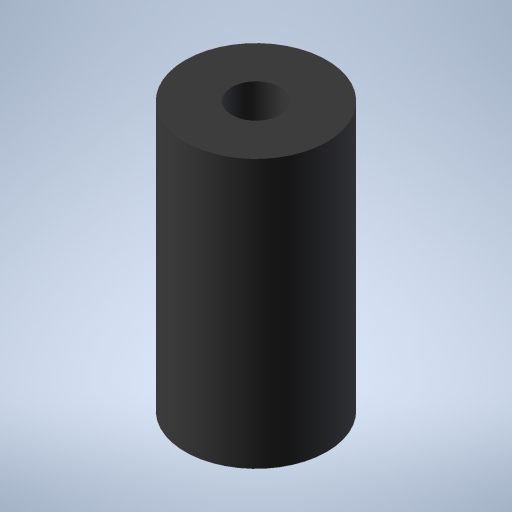
# Autodesk Inventor part: encoder_insert_2to6
Saved by Autodesk Inventor 2023 (Build 270158000, 158)
## iProperties
Created: 2023-04-28
Part Number: encoder_insert_2to6
Material: Generic
Document SubType Name: Modeling
Designer: jxl19
Density: 1 g/cm^3
Appearance: Default
Author: jxl19
## iProperties of the stored document encoder_insert_2to6_3DPrint.ipt
Created: 2023-04-28
Part Number: encoder_insert_2to6_3DPrint
Material: Generic
Document SubType Name: Modeling
Designer: jxl19
Density: 1 g/cm^3
Appearance: Default
Author: jxl19
Autodesk Inventor part; units mm, degrees
ref_plane "YZ Plane" through (0, 0, 0) normal (1, 0, 0) x (0, 1, 0)
ref_plane "XZ Plane" through (0, 0, 0) normal (0, 1, 0) x (-1, 0, 0)
ref_plane "XY Plane" through (0, 0, 0) normal (0, 0, 1) x (1, 0, 0)
sketch "Sketch1" plane through (0, 0, 0) normal (0, 1, 0) x (-1, 0, 0)
  circle A0 centre (0, 0) radius 2.9
  dimension "d0" = 5.8
  constraints: 1 centre point, 1 coincident
  measures "d0" diameter of A0
extrude "Extrusion1" add sketch "Sketch1" along normal blind 11
sketch "Sketch2" plane through (0, 11, 0) normal (0, 1, 0) x (1, 0, 0)
  circle A0 centre (0, 0) radius 1
  dimension "d3" = 2
  constraints: 1 centre point, 1 coincident
  measures "d3" diameter of A0
extrude "Extrusion2" cut sketch "Sketch2" against normal blind 10.7
body "Solid1"
